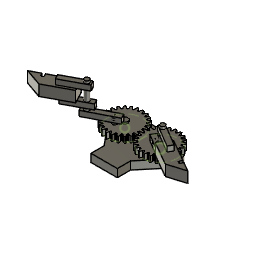
Manus Claw v1 (Autodesk Fusion 360 design; units mm, degrees)
description: Spur Gear; Module: 0.550000; Num Teeth: 24; Pressure Angle: 20.000000; Backlash: 0.00 mm
description: Spur Gear; Module: 0.5500000021653543; Num Teeth: 24; Pressure Angle: 20.0; Backlash: 0.00 mm
Autodesk Fusion 360 part; units mm, degrees
(part 1 of 11)
sketch "Sketch5" plane through (0, 0, 0) normal (0, 0, 1) x (1, 0, 0)
  line L0 (0, 0) -> (10, 0)
  line L1 (10, 0) -> (10, 5)
  line L2 (10, 5) -> (0, 5)
  line L3 (0, 5) -> (0, 0)
  line L4 (0, 5) -> (0, 10)
  line L5 (0, 10) -> (-8.1241, 19.7489)
  arc A0 (-7.2201, 22.9266) -> (-8.1241, 19.7489) centre (-6.5876, 21.0293) ccw
  line L6 (10, 5) -> (10, 10)
  line L7 (-7.2201, 22.9266) -> (-1.2199, 25.4807)
  line L8 (1.3259, 26) -> (5, 26)
  line L9 (0, 10) -> (10, 10)
  arc A1 (1.3259, 26) -> (-1.2199, 25.4807) centre (1.3259, 19.5) ccw
  line L10 (10, 10) -> (18.1241, 19.7489)
  line L11 (17.2201, 22.9266) -> (11.2199, 25.4807)
  line L12 (8.6741, 26) -> (5, 26)
  arc A2 (11.2199, 25.4807) -> (8.6741, 26) centre (8.6741, 19.5) ccw
  arc A3 (18.1241, 19.7489) -> (17.2201, 22.9266) centre (16.5876, 21.0293) ccw
  line L13 (10, 10) -> (0, 10)
  dimension "d15" = 2
  dimension "d24" = 6.5
  constraint horizontal L0
  constraint vertical L1
  constraint horizontal L2
  constraint vertical L3
  constraint coincident L0.start L3.end
  constraint perpendicular L2 L4
  constraint tangent L5 A0
  constraint horizontal L8
  constraint perpendicular L6 L9
  constraint tangent L7 A1
  constraint tangent L8 A1
  measures "d15" radius of A0
  measures "d24" radius of A1
extrude "Extrude5" add sketch "Sketch5" along normal blind 3 contours L2 L4 L6 L9 L13 | L5 A0 L7 L8 L9 A1 L10 L11 L12 A2 A3 L13 makes body 1
sketch "Sketch20" plane through (0, 0, 3) normal (0, 0, 1) x (-1, 0, 0)
  line L0 (-10, -5) -> (-10, -10)
  line L1 (-10, -10) -> (-18.1241, -19.7489)
  arc A0 (-18.1241, -19.7489) -> (-17.2201, -22.9266) centre (-16.5876, -21.0293) ccw
  line L2 (-17.2201, -22.9266) -> (-11.2199, -25.4807)
  arc A1 (-11.2199, -25.4807) -> (-8.6741, -26) centre (-8.6741, -19.5) ccw
  line L3 (-8.6741, -26) -> (-1.3259, -26)
  arc A2 (-1.3259, -26) -> (1.2199, -25.4807) centre (-1.3259, -19.5) ccw
  line L4 (1.2199, -25.4807) -> (7.2201, -22.9266)
  arc A3 (7.2201, -22.9266) -> (8.1241, -19.7489) centre (6.5876, -21.0293) ccw
  line L5 (8.1241, -19.7489) -> (0, -10)
  line L6 (0, -10) -> (0, -5)
  line L7 (0, -5) -> (-10, -5)
  line L8 (-5, -26) -> (-5, -5) construction
  circle A4 centre (1.6741, -19.5) radius 1.225
  circle A5 centre (-11.6741, -19.5) radius 1.225
  point P0 (-11.6741, -19.5)
  dimension "d136" = 2.45
  dimension "d137" = 2.45
  constraint midpoint L3 L8.start
  constraint midpoint L7 L8.end
  constraint symmetric L8 A4.centre P0
  constraint coincident P0 A5.centre
  measures "d136" diameter of A4
  measures "d137" diameter of A5
sketch "Sketch1" plane through (0, 0, 0) normal (0, 0, 1) x (1, 0, 0) in component "Spur Gear (24 teeth)"
  circle A0 centre (0, 0) radius 5.8892
  circle A1 centre (0, 0) radius 1.25
extrude "Extrude1" add sketch "Sketch1" along normal blind 2.2 separate body makes body 2 in component "Spur Gear (24 teeth)"
sketch "Sketch2" plane through (0, 0, 0) normal (0, 0, 1) x (1, 0, 0) in component "Spur Gear (24 teeth)"
  spline S0 degree 5 poles (6.182, -0.4978) (6.1847, -0.498) (6.1902, -0.4984) (6.1984, -0.4987) (6.2094, -0.4988) (6.2232, -0.4984) (6.2369, -0.4976) (6.2507, -0.4965) (6.2645, -0.4954) (6.2783, -0.4941) (6.2921, -0.4927) (6.306, -0.4912) (6.3198, -0.4895) (6.3336, -0.4877) (6.3475, -0.4857) (6.3613, -0.4835) (6.3752, -0.4811) (6.389, -0.4786) (6.4029, -0.476) (6.4168, -0.4733) (6.4306, -0.4705) (6.4445, -0.4676) (6.4583, -0.4646) (6.4722, -0.4615) (6.4861, -0.4582) (6.4999, -0.4548) (6.5138, -0.4514) (6.5277, -0.4478) (6.5415, -0.4441) (6.5554, -0.4403) (6.5693, -0.4364) (6.5831, -0.4325) (6.597, -0.4284) (6.6109, -0.4242) (6.6247, -0.42) (6.6386, -0.4156) (6.6524, -0.4112) (6.6663, -0.4067) (6.6801, -0.402) (6.694, -0.3973) (6.7078, -0.3925) (6.7216, -0.3877) (6.7355, -0.3827) (6.7493, -0.3776) (6.7631, -0.3725) (6.7769, -0.3673) (6.7907, -0.362) (6.8045, -0.3566) (6.8183, -0.3511) (6.8321, -0.3456) (6.8459, -0.3399) (6.8597, -0.3342) (6.8735, -0.3284) (6.8872, -0.3226) (6.901, -0.3166) (6.9147, -0.3106) (6.9285, -0.3045) (6.9422, -0.2983) (6.956, -0.2921) (6.9697, -0.2857) (6.9834, -0.2793) (6.9971, -0.2729) (7.0108, -0.2663) (7.0245, -0.2597) (7.0382, -0.253) (7.0519, -0.2462) (7.0655, -0.2394) (7.0792, -0.2324) (7.0928, -0.2254) (7.1064, -0.2184) (7.1201, -0.2113) (7.131, -0.2055) (7.1391, -0.2011) (7.1446, -0.1982) (7.1473, -0.1968) knots 0 0 0 0 0 0 0.01428571 0.02857143 0.04285714 0.05714286 0.07142857 0.08571429 0.1 0.11428571 0.12857143 0.14285714 0.15714286 0.17142857 0.18571429 0.2 0.21428571 0.22857143 0.24285714 0.25714286 0.27142857 0.28571429 0.3 0.31428571 0.32857143 0.34285714 0.35714286 0.37142857 0.38571429 0.4 0.41428571 0.42857143 0.44285714 0.45714286 0.47142857 0.48571429 0.5 0.51428571 0.52857143 0.54285714 0.55714286 0.57142857 0.58571429 0.6 0.61428571 0.62857143 0.64285714 0.65714286 0.67142857 0.68571429 0.7 0.71428571 0.72857143 0.74285714 0.75714286 0.77142857 0.78571429 0.8 0.81428571 0.82857143 0.84285714 0.85714286 0.87142857 0.88571429 0.9 0.91428571 0.92857143 0.94285714 0.95714286 0.97142857 0.98571429 1 1 1 1 1 1
  spline S1 degree 5 poles (6.182, 0.4978) (6.1847, 0.498) (6.1902, 0.4984) (6.1984, 0.4987) (6.2094, 0.4988) (6.2232, 0.4984) (6.2369, 0.4976) (6.2507, 0.4965) (6.2645, 0.4954) (6.2783, 0.4941) (6.2921, 0.4927) (6.306, 0.4912) (6.3198, 0.4895) (6.3336, 0.4877) (6.3475, 0.4857) (6.3613, 0.4835) (6.3752, 0.4811) (6.389, 0.4786) (6.4029, 0.476) (6.4168, 0.4733) (6.4306, 0.4705) (6.4445, 0.4676) (6.4583, 0.4646) (6.4722, 0.4615) (6.4861, 0.4582) (6.4999, 0.4548) (6.5138, 0.4514) (6.5277, 0.4478) (6.5415, 0.4441) (6.5554, 0.4403) (6.5693, 0.4364) (6.5831, 0.4325) (6.597, 0.4284) (6.6109, 0.4242) (6.6247, 0.42) (6.6386, 0.4156) (6.6524, 0.4112) (6.6663, 0.4067) (6.6801, 0.402) (6.694, 0.3973) (6.7078, 0.3925) (6.7216, 0.3877) (6.7355, 0.3827) (6.7493, 0.3776) (6.7631, 0.3725) (6.7769, 0.3673) (6.7907, 0.362) (6.8045, 0.3566) (6.8183, 0.3511) (6.8321, 0.3456) (6.8459, 0.3399) (6.8597, 0.3342) (6.8735, 0.3284) (6.8872, 0.3226) (6.901, 0.3166) (6.9147, 0.3106) (6.9285, 0.3045) (6.9422, 0.2983) (6.956, 0.2921) (6.9697, 0.2857) (6.9834, 0.2793) (6.9971, 0.2729) (7.0108, 0.2663) (7.0245, 0.2597) (7.0382, 0.253) (7.0519, 0.2462) (7.0655, 0.2394) (7.0792, 0.2324) (7.0928, 0.2254) (7.1064, 0.2184) (7.1201, 0.2113) (7.131, 0.2055) (7.1391, 0.2011) (7.1446, 0.1982) (7.1473, 0.1968) knots 0 0 0 0 0 0 0.01428571 0.02857143 0.04285714 0.05714286 0.07142857 0.08571429 0.1 0.11428571 0.12857143 0.14285714 0.15714286 0.17142857 0.18571429 0.2 0.21428571 0.22857143 0.24285714 0.25714286 0.27142857 0.28571429 0.3 0.31428571 0.32857143 0.34285714 0.35714286 0.37142857 0.38571429 0.4 0.41428571 0.42857143 0.44285714 0.45714286 0.47142857 0.48571429 0.5 0.51428571 0.52857143 0.54285714 0.55714286 0.57142857 0.58571429 0.6 0.61428571 0.62857143 0.64285714 0.65714286 0.67142857 0.68571429 0.7 0.71428571 0.72857143 0.74285714 0.75714286 0.77142857 0.78571429 0.8 0.81428571 0.82857143 0.84285714 0.85714286 0.87142857 0.88571429 0.9 0.91428571 0.92857143 0.94285714 0.95714286 0.97142857 0.98571429 1 1 1 1 1 1
  arc A0 (7.1473, -0.1968) -> (7.1473, 0.1968) centre (0, 0) ccw
  line L0 (5.8602, -0.4727) -> (6.182, -0.4978)
  line L1 (5.8602, 0.4727) -> (6.182, 0.4978)
  line L2 (5.8602, -0.4727) -> (5.8602, 0.4727)
  point P0 (6.25, -0.4966)
  point P1 (6.3185, -0.4897)
  point P2 (6.3872, -0.4789)
  point P3 (6.4561, -0.4651)
  point P4 (6.5252, -0.4484)
  point P5 (6.5943, -0.4292)
  point P6 (6.6635, -0.4075)
  point P7 (6.7328, -0.3836)
  point P8 (6.802, -0.3575)
  point P9 (6.8712, -0.3294)
  point P10 (6.9404, -0.2991)
  point P11 (7.0095, -0.2669)
  point P12 (7.0785, -0.2328)
  point P13 (6.25, 0.4966)
  point P14 (6.3185, 0.4897)
  point P15 (6.3872, 0.4789)
  point P16 (6.4561, 0.4651)
  point P17 (6.5252, 0.4484)
  point P18 (6.5943, 0.4292)
  point P19 (6.6635, 0.4075)
  point P20 (6.7328, 0.3836)
  point P21 (6.802, 0.3575)
  point P22 (6.8712, 0.3294)
  point P23 (6.9404, 0.2991)
  point P24 (7.0095, 0.2669)
  point P25 (7.0785, 0.2328)
extrude "Extrude2" add sketch "Sketch2" along normal blind 2.2 bodies 2 in component "Spur Gear (24 teeth)"
fillet "Fillet1" radius 0.25 2 edges at (5.8701, -0.4735, 1.1) (5.8701, 0.4735, 1.1) on bodies 2 in component "Spur Gear (24 teeth)"
pattern_circular "C-Pattern1" count 24 over 360 about axis through (0, 0, 0) along (0, 0, 1) of "Extrude2", "Fillet1" in component "Spur Gear (24 teeth)"
sketch "Sketch3" plane through (0, 0, 0) normal (0, 0, 1) x (1, 0, 0) in component "Spur Gear (24 teeth)"
  circle A0 centre (0, 0) radius 6.6 construction
extrude "Extrude16" add sketch "Sketch20" along normal blind 3 contours A4 | A5 bodies 1
sketch "Sketch1 (2)" plane through (0, 0, 0) normal (0, 0, 1) x (1, 0, 0) in component "Spur Gear (24 teeth) (1)"
  circle A0 centre (0, 0) radius 5.8892
  circle A1 centre (0, 0) radius 1.25
extrude "Extrude1'" add sketch "Sketch1 (2)" along normal blind 2.2 separate body makes body 3 in component "Spur Gear (24 teeth) (1)"
sketch "Sketch2 (2)" plane through (0, 0, 0) normal (0, 0, 1) x (1, 0, 0) in component "Spur Gear (24 teeth) (1)"
  spline S0 degree 5 poles (6.182, -0.4978) (6.1847, -0.498) (6.1902, -0.4984) (6.1984, -0.4987) (6.2094, -0.4988) (6.2232, -0.4984) (6.2369, -0.4976) (6.2507, -0.4965) (6.2645, -0.4954) (6.2783, -0.4941) (6.2921, -0.4927) (6.306, -0.4912) (6.3198, -0.4895) (6.3336, -0.4877) (6.3475, -0.4857) (6.3613, -0.4835) (6.3752, -0.4811) (6.389, -0.4786) (6.4029, -0.476) (6.4168, -0.4733) (6.4306, -0.4705) (6.4445, -0.4676) (6.4583, -0.4646) (6.4722, -0.4615) (6.4861, -0.4582) (6.4999, -0.4548) (6.5138, -0.4514) (6.5277, -0.4478) (6.5415, -0.4441) (6.5554, -0.4403) (6.5693, -0.4364) (6.5831, -0.4325) (6.597, -0.4284) (6.6109, -0.4242) (6.6247, -0.42) (6.6386, -0.4156) (6.6524, -0.4112) (6.6663, -0.4067) (6.6801, -0.402) (6.694, -0.3973) (6.7078, -0.3925) (6.7216, -0.3877) (6.7355, -0.3827) (6.7493, -0.3776) (6.7631, -0.3725) (6.7769, -0.3673) (6.7907, -0.362) (6.8045, -0.3566) (6.8183, -0.3511) (6.8321, -0.3456) (6.8459, -0.3399) (6.8597, -0.3342) (6.8735, -0.3284) (6.8872, -0.3226) (6.901, -0.3166) (6.9147, -0.3106) (6.9285, -0.3045) (6.9422, -0.2983) (6.956, -0.2921) (6.9697, -0.2857) (6.9834, -0.2793) (6.9971, -0.2729) (7.0108, -0.2663) (7.0245, -0.2597) (7.0382, -0.253) (7.0519, -0.2462) (7.0655, -0.2394) (7.0792, -0.2324) (7.0928, -0.2254) (7.1064, -0.2184) (7.1201, -0.2113) (7.131, -0.2055) (7.1391, -0.2011) (7.1446, -0.1982) (7.1473, -0.1968) knots 0 0 0 0 0 0 0.01428571 0.02857143 0.04285714 0.05714286 0.07142857 0.08571429 0.1 0.11428571 0.12857143 0.14285714 0.15714286 0.17142857 0.18571429 0.2 0.21428571 0.22857143 0.24285714 0.25714286 0.27142857 0.28571429 0.3 0.31428571 0.32857143 0.34285714 0.35714286 0.37142857 0.38571429 0.4 0.41428571 0.42857143 0.44285714 0.45714286 0.47142857 0.48571429 0.5 0.51428571 0.52857143 0.54285714 0.55714286 0.57142857 0.58571429 0.6 0.61428571 0.62857143 0.64285714 0.65714286 0.67142857 0.68571429 0.7 0.71428571 0.72857143 0.74285714 0.75714286 0.77142857 0.78571429 0.8 0.81428571 0.82857143 0.84285714 0.85714286 0.87142857 0.88571429 0.9 0.91428571 0.92857143 0.94285714 0.95714286 0.97142857 0.98571429 1 1 1 1 1 1
  spline S1 degree 5 poles (6.182, 0.4978) (6.1847, 0.498) (6.1902, 0.4984) (6.1984, 0.4987) (6.2094, 0.4988) (6.2232, 0.4984) (6.2369, 0.4976) (6.2507, 0.4965) (6.2645, 0.4954) (6.2783, 0.4941) (6.2921, 0.4927) (6.306, 0.4912) (6.3198, 0.4895) (6.3336, 0.4877) (6.3475, 0.4857) (6.3613, 0.4835) (6.3752, 0.4811) (6.389, 0.4786) (6.4029, 0.476) (6.4168, 0.4733) (6.4306, 0.4705) (6.4445, 0.4676) (6.4583, 0.4646) (6.4722, 0.4615) (6.4861, 0.4582) (6.4999, 0.4548) (6.5138, 0.4514) (6.5277, 0.4478) (6.5415, 0.4441) (6.5554, 0.4403) (6.5693, 0.4364) (6.5831, 0.4325) (6.597, 0.4284) (6.6109, 0.4242) (6.6247, 0.42) (6.6386, 0.4156) (6.6524, 0.4112) (6.6663, 0.4067) (6.6801, 0.402) (6.694, 0.3973) (6.7078, 0.3925) (6.7216, 0.3877) (6.7355, 0.3827) (6.7493, 0.3776) (6.7631, 0.3725) (6.7769, 0.3673) (6.7907, 0.362) (6.8045, 0.3566) (6.8183, 0.3511) (6.8321, 0.3456) (6.8459, 0.3399) (6.8597, 0.3342) (6.8735, 0.3284) (6.8872, 0.3226) (6.901, 0.3166) (6.9147, 0.3106) (6.9285, 0.3045) (6.9422, 0.2983) (6.956, 0.2921) (6.9697, 0.2857) (6.9834, 0.2793) (6.9971, 0.2729) (7.0108, 0.2663) (7.0245, 0.2597) (7.0382, 0.253) (7.0519, 0.2462) (7.0655, 0.2394) (7.0792, 0.2324) (7.0928, 0.2254) (7.1064, 0.2184) (7.1201, 0.2113) (7.131, 0.2055) (7.1391, 0.2011) (7.1446, 0.1982) (7.1473, 0.1968) knots 0 0 0 0 0 0 0.01428571 0.02857143 0.04285714 0.05714286 0.07142857 0.08571429 0.1 0.11428571 0.12857143 0.14285714 0.15714286 0.17142857 0.18571429 0.2 0.21428571 0.22857143 0.24285714 0.25714286 0.27142857 0.28571429 0.3 0.31428571 0.32857143 0.34285714 0.35714286 0.37142857 0.38571429 0.4 0.41428571 0.42857143 0.44285714 0.45714286 0.47142857 0.48571429 0.5 0.51428571 0.52857143 0.54285714 0.55714286 0.57142857 0.58571429 0.6 0.61428571 0.62857143 0.64285714 0.65714286 0.67142857 0.68571429 0.7 0.71428571 0.72857143 0.74285714 0.75714286 0.77142857 0.78571429 0.8 0.81428571 0.82857143 0.84285714 0.85714286 0.87142857 0.88571429 0.9 0.91428571 0.92857143 0.94285714 0.95714286 0.97142857 0.98571429 1 1 1 1 1 1
  arc A0 (7.1473, -0.1968) -> (7.1473, 0.1968) centre (0, 0) ccw
  line L0 (5.8602, -0.4727) -> (6.182, -0.4978)
  line L1 (5.8602, 0.4727) -> (6.182, 0.4978)
  line L2 (5.8602, -0.4727) -> (5.8602, 0.4727)
  point P0 (6.25, -0.4966)
  point P1 (6.3185, -0.4897)
  point P2 (6.3872, -0.4789)
  point P3 (6.4561, -0.4651)
  point P4 (6.5252, -0.4484)
  point P5 (6.5943, -0.4292)
  point P6 (6.6635, -0.4075)
  point P7 (6.7328, -0.3836)
  point P8 (6.802, -0.3575)
  point P9 (6.8712, -0.3294)
  point P10 (6.9404, -0.2991)
  point P11 (7.0095, -0.2669)
  point P12 (7.0785, -0.2328)
  point P13 (6.25, 0.4966)
  point P14 (6.3185, 0.4897)
  point P15 (6.3872, 0.4789)
  point P16 (6.4561, 0.4651)
  point P17 (6.5252, 0.4484)
  point P18 (6.5943, 0.4292)
  point P19 (6.6635, 0.4075)
  point P20 (6.7328, 0.3836)
  point P21 (6.802, 0.3575)
  point P22 (6.8712, 0.3294)
  point P23 (6.9404, 0.2991)
  point P24 (7.0095, 0.2669)
  point P25 (7.0785, 0.2328)
extrude "Extrude2'" add sketch "Sketch2 (2)" along normal blind 2.2 bodies 3 in component "Spur Gear (24 teeth) (1)"
fillet "Fillet1'" radius 0.25 2 edges at (5.8701, -0.4735, 1.1) (5.8701, 0.4735, 1.1) on bodies 3 in component "Spur Gear (24 teeth) (1)"
pattern_circular "C-Pattern1'" count 24 over 360 about axis through (0, 0, 0) along (0, 0, 1) of "Extrude2'", "Fillet1'" in component "Spur Gear (24 teeth) (1)"
sketch "Sketch3 (2)" plane through (0, 0, 0) normal (0, 0, 1) x (1, 0, 0) in component "Spur Gear (24 teeth) (1)"
  circle A0 centre (0, 0) radius 6.6 construction
sketch "Sketch21" plane through (30.0306, 32.9006, 5.45) normal (0, 0, 1) x (0.920765, -0.390118, 0)
  arc A0 (-5.983, -17.9856) -> (-6.0137, -17.8745) centre (-11.6741, -19.5) ccw
  arc A1 (-5.8527, -17.5684) -> (-6.0137, -17.8745) centre (-5.7734, -17.8055) ccw
  line L0 (-5.8527, -17.5684) -> (-5.7878, -17.5467)
  spline S0 degree 5 poles (-5.7878, -17.5467) (-5.7852, -17.5458) (-5.78, -17.544) (-5.7723, -17.5411) (-5.7621, -17.5369) (-5.7496, -17.5311) (-5.7373, -17.525) (-5.725, -17.5187) (-5.7127, -17.5122) (-5.7005, -17.5056) (-5.6883, -17.499) (-5.6762, -17.4922) (-5.6641, -17.4853) (-5.6521, -17.4782) (-5.6401, -17.4709) (-5.6282, -17.4635) (-5.6164, -17.4559) (-5.6046, -17.4482) (-5.5929, -17.4404) (-5.5812, -17.4326) (-5.5695, -17.4246) (-5.5579, -17.4165) (-5.5463, -17.4083) (-5.5347, -17.4) (-5.5232, -17.3916) (-5.5118, -17.3831) (-5.5004, -17.3744) (-5.489, -17.3657) (-5.4777, -17.3569) (-5.4664, -17.3481) (-5.4551, -17.3391) (-5.4439, -17.33) (-5.4327, -17.3209) (-5.4216, -17.3116) (-5.4105, -17.3023) (-5.3994, -17.2929) (-5.3884, -17.2834) (-5.3774, -17.2738) (-5.3665, -17.2642) (-5.3556, -17.2544) (-5.3447, -17.2446) (-5.3339, -17.2347) (-5.3231, -17.2247) (-5.3123, -17.2147) (-5.3016, -17.2046) (-5.2909, -17.1944) (-5.2803, -17.1841) (-5.2697, -17.1738) (-5.2591, -17.1633) (-5.2486, -17.1529) (-5.2381, -17.1423) (-5.2276, -17.1317) (-5.2172, -17.121) (-5.2068, -17.1102) (-5.1964, -17.0993) (-5.1861, -17.0884) (-5.1758, -17.0774) (-5.1656, -17.0664) (-5.1554, -17.0553) (-5.1452, -17.0441) (-5.1351, -17.0329) (-5.125, -17.0215) (-5.1149, -17.0102) (-5.1049, -16.9987) (-5.0949, -16.9872) (-5.085, -16.9756) (-5.0751, -16.964) (-5.0652, -16.9523) (-5.0554, -16.9406) (-5.0456, -16.9287) (-5.0358, -16.9168) (-5.028, -16.9073) (-5.0222, -16.9001) (-5.0183, -16.8953) (-5.0164, -16.8929) knots 0 0 0 0 0 0 0.01428571 0.02857143 0.04285714 0.05714286 0.07142857 0.08571429 0.1 0.11428571 0.12857143 0.14285714 0.15714286 0.17142857 0.18571429 0.2 0.21428571 0.22857143 0.24285714 0.25714286 0.27142857 0.28571429 0.3 0.31428571 0.32857143 0.34285714 0.35714286 0.37142857 0.38571429 0.4 0.41428571 0.42857143 0.44285714 0.45714286 0.47142857 0.48571429 0.5 0.51428571 0.52857143 0.54285714 0.55714286 0.57142857 0.58571429 0.6 0.61428571 0.62857143 0.64285714 0.65714286 0.67142857 0.68571429 0.7 0.71428571 0.72857143 0.74285714 0.75714286 0.77142857 0.78571429 0.8 0.81428571 0.82857143 0.84285714 0.85714286 0.87142857 0.88571429 0.9 0.91428571 0.92857143 0.94285714 0.95714286 0.97142857 0.98571429 1 1 1 1 1 1
  arc A2 (-5.0164, -16.8929) -> (-5.1699, -16.5306) centre (-11.6741, -19.5) ccw
  spline S1 degree 5 poles (-5.1699, -16.5306) (-5.173, -16.5303) (-5.1791, -16.5297) (-5.1884, -16.5289) (-5.2006, -16.5278) (-5.216, -16.5266) (-5.2313, -16.5254) (-5.2466, -16.5243) (-5.2618, -16.5232) (-5.2771, -16.5223) (-5.2923, -16.5213) (-5.3075, -16.5205) (-5.3227, -16.5198) (-5.3379, -16.5191) (-5.353, -16.5184) (-5.3682, -16.5179) (-5.3833, -16.5174) (-5.3984, -16.517) (-5.4134, -16.5167) (-5.4285, -16.5164) (-5.4435, -16.5163) (-5.4585, -16.5162) (-5.4734, -16.5161) (-5.4884, -16.5162) (-5.5033, -16.5163) (-5.5182, -16.5165) (-5.533, -16.5168) (-5.5479, -16.5171) (-5.5627, -16.5175) (-5.5775, -16.518) (-5.5922, -16.5186) (-5.607, -16.5193) (-5.6217, -16.52) (-5.6363, -16.5208) (-5.651, -16.5217) (-5.6656, -16.5227) (-5.6802, -16.5238) (-5.6947, -16.5249) (-5.7092, -16.5262) (-5.7237, -16.5275) (-5.7382, -16.5289) (-5.7526, -16.5304) (-5.767, -16.5319) (-5.7813, -16.5336) (-5.7956, -16.5353) (-5.8099, -16.5372) (-5.8242, -16.5391) (-5.8384, -16.5411) (-5.8525, -16.5432) (-5.8667, -16.5455) (-5.8807, -16.5478) (-5.8948, -16.5502) (-5.9088, -16.5527) (-5.9227, -16.5553) (-5.9366, -16.558) (-5.9505, -16.5609) (-5.9643, -16.5638) (-5.9781, -16.5668) (-5.9918, -16.5699) (-6.0055, -16.5732) (-6.0191, -16.5765) (-6.0326, -16.5801) (-6.0461, -16.5838) (-6.0594, -16.5877) (-6.0728, -16.5917) (-6.086, -16.5958) (-6.0992, -16.6) (-6.1124, -16.6043) (-6.1255, -16.6087) (-6.1385, -16.6133) (-6.1513, -16.6183) (-6.1614, -16.6227) (-6.1689, -16.6262) (-6.1738, -16.6287) (-6.1762, -16.6299) knots -1 -1 -1 -1 -1 -1 -0.98571429 -0.97142857 -0.95714286 -0.94285714 -0.92857143 -0.91428571 -0.9 -0.88571429 -0.87142857 -0.85714286 -0.84285714 -0.82857143 -0.81428571 -0.8 -0.78571429 -0.77142857 -0.75714286 -0.74285714 -0.72857143 -0.71428571 -0.7 -0.68571429 -0.67142857 -0.65714286 -0.64285714 -0.62857143 -0.61428571 -0.6 -0.58571429 -0.57142857 -0.55714286 -0.54285714 -0.52857143 -0.51428571 -0.5 -0.48571429 -0.47142857 -0.45714286 -0.44285714 -0.42857143 -0.41428571 -0.4 -0.38571429 -0.37142857 -0.35714286 -0.34285714 -0.32857143 -0.31428571 -0.3 -0.28571429 -0.27142857 -0.25714286 -0.24285714 -0.22857143 -0.21428571 -0.2 -0.18571429 -0.17142857 -0.15714286 -0.14285714 -0.12857143 -0.11428571 -0.1 -0.08571429 -0.07142857 -0.05714286 -0.04285714 -0.02857143 -0.01428571 0 0 0 0 0 0
  line L1 (-6.1762, -16.6299) -> (-6.237, -16.6615)
  arc A3 (-6.5689, -16.5642) -> (-6.237, -16.6615) centre (-6.3521, -16.4396) ccw
  arc A4 (-6.5689, -16.5642) -> (-6.6273, -16.4649) centre (-11.6741, -19.5) ccw
  arc A5 (-6.551, -16.1275) -> (-6.6273, -16.4649) centre (-6.4131, -16.336) ccw
  line L2 (-6.551, -16.1275) -> (-6.4939, -16.0897)
  spline S2 degree 5 poles (-6.4939, -16.0897) (-6.4916, -16.0882) (-6.4871, -16.0851) (-6.4804, -16.0803) (-6.4717, -16.0737) (-6.4611, -16.0649) (-6.4507, -16.0558) (-6.4405, -16.0464) (-6.4304, -16.037) (-6.4203, -16.0275) (-6.4102, -16.0179) (-6.4002, -16.0082) (-6.3903, -15.9984) (-6.3806, -15.9885) (-6.3709, -15.9783) (-6.3613, -15.9681) (-6.3519, -15.9577) (-6.3425, -15.9472) (-6.3331, -15.9367) (-6.3239, -15.926) (-6.3147, -15.9153) (-6.3055, -15.9045) (-6.2964, -15.8936) (-6.2874, -15.8825) (-6.2785, -15.8714) (-6.2697, -15.8603) (-6.2609, -15.849) (-6.2521, -15.8376) (-6.2435, -15.8262) (-6.2349, -15.8147) (-6.2263, -15.8031) (-6.2178, -15.7914) (-6.2094, -15.7797) (-6.201, -15.7679) (-6.1927, -15.756) (-6.1845, -15.7441) (-6.1763, -15.7321) (-6.1682, -15.72) (-6.1601, -15.7078) (-6.1521, -15.6956) (-6.1441, -15.6833) (-6.1362, -15.6709) (-6.1284, -15.6585) (-6.1206, -15.646) (-6.1128, -15.6335) (-6.1052, -15.6208) (-6.0975, -15.6082) (-6.09, -15.5954) (-6.0824, -15.5826) (-6.075, -15.5698) (-6.0676, -15.5568) (-6.0602, -15.5439) (-6.0529, -15.5308) (-6.0457, -15.5177) (-6.0385, -15.5046) (-6.0313, -15.4914) (-6.0243, -15.4781) (-6.0172, -15.4648) (-6.0103, -15.4514) (-6.0033, -15.438) (-5.9964, -15.4245) (-5.9896, -15.411) (-5.9829, -15.3974) (-5.9761, -15.3837) (-5.9695, -15.37) (-5.9629, -15.3563) (-5.9563, -15.3425) (-5.9498, -15.3286) (-5.9433, -15.3147) (-5.9369, -15.3007) (-5.9306, -15.2867) (-5.9255, -15.2755) (-5.9218, -15.267) (-5.9193, -15.2614) (-5.918, -15.2586) knots 0 0 0 0 0 0 0.01428571 0.02857143 0.04285714 0.05714286 0.07142857 0.08571429 0.1 0.11428571 0.12857143 0.14285714 0.15714286 0.17142857 0.18571429 0.2 0.21428571 0.22857143 0.24285714 0.25714286 0.27142857 0.28571429 0.3 0.31428571 0.32857143 0.34285714 0.35714286 0.37142857 0.38571429 0.4 0.41428571 0.42857143 0.44285714 0.45714286 0.47142857 0.48571429 0.5 0.51428571 0.52857143 0.54285714 0.55714286 0.57142857 0.58571429 0.6 0.61428571 0.62857143 0.64285714 0.65714286 0.67142857 0.68571429 0.7 0.71428571 0.72857143 0.74285714 0.75714286 0.77142857 0.78571429 0.8 0.81428571 0.82857143 0.84285714 0.85714286 0.87142857 0.88571429 0.9 0.91428571 0.92857143 0.94285714 0.95714286 0.97142857 0.98571429 1 1 1 1 1 1
  arc A6 (-5.918, -15.2586) -> (-6.1601, -14.9483) centre (-11.6741, -19.5) ccw
  spline S3 degree 5 poles (-6.1601, -14.9483) (-6.1631, -14.9488) (-6.1692, -14.9499) (-6.1783, -14.9515) (-6.1905, -14.9536) (-6.2056, -14.9564) (-6.2207, -14.9592) (-6.2358, -14.9621) (-6.2508, -14.965) (-6.2658, -14.968) (-6.2807, -14.9711) (-6.2956, -14.9742) (-6.3105, -14.9774) (-6.3253, -14.9807) (-6.3401, -14.984) (-6.3549, -14.9874) (-6.3696, -14.9909) (-6.3843, -14.9944) (-6.3989, -14.998) (-6.4135, -15.0016) (-6.428, -15.0053) (-6.4425, -15.0091) (-6.457, -15.0129) (-6.4714, -15.0168) (-6.4858, -15.0208) (-6.5001, -15.0249) (-6.5144, -15.029) (-6.5287, -15.0332) (-6.5429, -15.0374) (-6.557, -15.0417) (-6.5711, -15.0461) (-6.5852, -15.0505) (-6.5992, -15.0551) (-6.6131, -15.0597) (-6.627, -15.0643) (-6.6409, -15.069) (-6.6547, -15.0738) (-6.6685, -15.0787) (-6.6822, -15.0837) (-6.6958, -15.0887) (-6.7094, -15.0938) (-6.723, -15.0989) (-6.7365, -15.1042) (-6.7499, -15.1095) (-6.7633, -15.1149) (-6.7766, -15.1204) (-6.7898, -15.1259) (-6.803, -15.1315) (-6.8162, -15.1373) (-6.8292, -15.143) (-6.8422, -15.1489) (-6.8552, -15.1549) (-6.868, -15.1609) (-6.8808, -15.1671) (-6.8936, -15.1733) (-6.9062, -15.1796) (-6.9188, -15.186) (-6.9313, -15.1925) (-6.9438, -15.1991) (-6.9561, -15.2057) (-6.9684, -15.2125) (-6.9806, -15.2194) (-6.9926, -15.2265) (-7.0045, -15.2337) (-7.0164, -15.241) (-7.0281, -15.2484) (-7.0398, -15.2559) (-7.0514, -15.2635) (-7.0629, -15.2711) (-7.0743, -15.279) (-7.0854, -15.2871) (-7.094, -15.2939) (-7.1002, -15.2993) (-7.1043, -15.3029) (-7.1064, -15.3048) knots -1 -1 -1 -1 -1 -1 -0.98571429 -0.97142857 -0.95714286 -0.94285714 -0.92857143 -0.91428571 -0.9 -0.88571429 -0.87142857 -0.85714286 -0.84285714 -0.82857143 -0.81428571 -0.8 -0.78571429 -0.77142857 -0.75714286 -0.74285714 -0.72857143 -0.71428571 -0.7 -0.68571429 -0.67142857 -0.65714286 -0.64285714 -0.62857143 -0.61428571 -0.6 -0.58571429 -0.57142857 -0.55714286 -0.54285714 -0.52857143 -0.51428571 -0.5 -0.48571429 -0.47142857 -0.45714286 -0.44285714 -0.42857143 -0.41428571 -0.4 -0.38571429 -0.37142857 -0.35714286 -0.34285714 -0.32857143 -0.31428571 -0.3 -0.28571429 -0.27142857 -0.25714286 -0.24285714 -0.22857143 -0.21428571 -0.2 -0.18571429 -0.17142857 -0.15714286 -0.14285714 -0.12857143 -0.11428571 -0.1 -0.08571429 -0.07142857 -0.05714286 -0.04285714 -0.02857143 -0.01428571 0 0 0 0 0 0
  line L3 (-7.1064, -15.3048) -> (-7.1569, -15.351)
  arc A7 (-7.5027, -15.3429) -> (-7.1569, -15.351) centre (-7.3256, -15.1664) ccw
  arc A8 (-7.5027, -15.3429) -> (-7.5848, -15.2621) centre (-11.6741, -19.5) ccw
  arc A9 (-7.5985, -14.9165) -> (-7.5848, -15.2621) centre (-7.4112, -15.0822) ccw
  line L4 (-7.5985, -14.9165) -> (-7.5531, -14.8652)
  spline S4 degree 5 poles (-7.5531, -14.8652) (-7.5513, -14.8631) (-7.5477, -14.859) (-7.5424, -14.8526) (-7.5357, -14.8439) (-7.5278, -14.8327) (-7.5201, -14.8212) (-7.5127, -14.8096) (-7.5053, -14.7978) (-7.498, -14.786) (-7.4908, -14.7742) (-7.4837, -14.7622) (-7.4767, -14.7502) (-7.4698, -14.738) (-7.4631, -14.7258) (-7.4565, -14.7134) (-7.45, -14.7009) (-7.4437, -14.6884) (-7.4374, -14.6757) (-7.4312, -14.663) (-7.4251, -14.6503) (-7.419, -14.6375) (-7.4131, -14.6246) (-7.4073, -14.6116) (-7.4015, -14.5986) (-7.3958, -14.5855) (-7.3903, -14.5723) (-7.3848, -14.5591) (-7.3794, -14.5458) (-7.374, -14.5325) (-7.3688, -14.5191) (-7.3636, -14.5056) (-7.3585, -14.4921) (-7.3535, -14.4785) (-7.3485, -14.4649) (-7.3436, -14.4512) (-7.3388, -14.4375) (-7.3341, -14.4237) (-7.3295, -14.4099) (-7.3249, -14.396) (-7.3204, -14.3821) (-7.3159, -14.3681) (-7.3116, -14.354) (-7.3073, -14.34) (-7.3031, -14.3258) (-7.2989, -14.3117) (-7.2948, -14.2974) (-7.2908, -14.2832) (-7.2869, -14.2689) (-7.283, -14.2545) (-7.2792, -14.2401) (-7.2754, -14.2257) (-7.2718, -14.2112) (-7.2682, -14.1967) (-7.2646, -14.1821) (-7.2611, -14.1675) (-7.2577, -14.1529) (-7.2544, -14.1382) (-7.2511, -14.1234) (-7.2479, -14.1087) (-7.2447, -14.0939) (-7.2416, -14.079) (-7.2386, -14.0641) (-7.2357, -14.0492) (-7.2328, -14.0343) (-7.2299, -14.0193) (-7.2272, -14.0042) (-7.2245, -13.9892) (-7.2218, -13.9741) (-7.2193, -13.9589) (-7.2168, -13.9438) (-7.2148, -13.9316) (-7.2134, -13.9225) (-7.2124, -13.9164) (-7.2119, -13.9133) knots 0 0 0 0 0 0 0.01428571 0.02857143 0.04285714 0.05714286 0.07142857 0.08571429 0.1 0.11428571 0.12857143 0.14285714 0.15714286 0.17142857 0.18571429 0.2 0.21428571 0.22857143 0.24285714 0.25714286 0.27142857 0.28571429 0.3 0.31428571 0.32857143 0.34285714 0.35714286 0.37142857 0.38571429 0.4 0.41428571 0.42857143 0.44285714 0.45714286 0.47142857 0.48571429 0.5 0.51428571 0.52857143 0.54285714 0.55714286 0.57142857 0.58571429 0.6 0.61428571 0.62857143 0.64285714 0.65714286 0.67142857 0.68571429 0.7 0.71428571 0.72857143 0.74285714 0.75714286 0.77142857 0.78571429 0.8 0.81428571 0.82857143 0.84285714 0.85714286 0.87142857 0.88571429 0.9 0.91428571 0.92857143 0.94285714 0.95714286 0.97142857 0.98571429 1 1 1 1 1 1
  arc A10 (-7.2119, -13.9133) -> (-7.526, -13.6763) centre (-11.6741, -19.5) ccw
  spline S5 degree 5 poles (-7.526, -13.6763) (-7.5288, -13.6776) (-7.5345, -13.6802) (-7.5428, -13.684) (-7.554, -13.6893) (-7.5679, -13.6958) (-7.5818, -13.7025) (-7.5956, -13.7092) (-7.6093, -13.7159) (-7.623, -13.7227) (-7.6366, -13.7295) (-7.6502, -13.7364) (-7.6638, -13.7433) (-7.6773, -13.7503) (-7.6907, -13.7574) (-7.7041, -13.7644) (-7.7174, -13.7716) (-7.7306, -13.7788) (-7.7438, -13.786) (-7.757, -13.7933) (-7.7701, -13.8007) (-7.7831, -13.8081) (-7.7961, -13.8155) (-7.809, -13.823) (-7.8219, -13.8306) (-7.8347, -13.8382) (-7.8474, -13.8459) (-7.8601, -13.8536) (-7.8727, -13.8614) (-7.8853, -13.8692) (-7.8977, -13.8771) (-7.9102, -13.885) (-7.9225, -13.893) (-7.9348, -13.9011) (-7.9471, -13.9092) (-7.9592, -13.9173) (-7.9713, -13.9255) (-7.9833, -13.9338) (-7.9953, -13.9421) (-8.0072, -13.9505) (-8.019, -13.9589) (-8.0308, -13.9674) (-8.0424, -13.976) (-8.054, -13.9846) (-8.0655, -13.9933) (-8.077, -14.002) (-8.0884, -14.0108) (-8.0996, -14.0197) (-8.1109, -14.0286) (-8.122, -14.0375) (-8.133, -14.0466) (-8.144, -14.0557) (-8.1548, -14.0649) (-8.1656, -14.0741) (-8.1763, -14.0834) (-8.1869, -14.0928) (-8.1974, -14.1022) (-8.2078, -14.1117) (-8.2181, -14.1213) (-8.2283, -14.131) (-8.2384, -14.1407) (-8.2484, -14.1505) (-8.2582, -14.1605) (-8.2678, -14.1705) (-8.2774, -14.1806) (-8.2868, -14.1908) (-8.2961, -14.2011) (-8.3054, -14.2114) (-8.3145, -14.2217) (-8.3235, -14.2323) (-8.3321, -14.243) (-8.3387, -14.2518) (-8.3433, -14.2586) (-8.3463, -14.2632) (-8.3478, -14.2655) knots -1 -1 -1 -1 -1 -1 -0.98571429 -0.97142857 -0.95714286 -0.94285714 -0.92857143 -0.91428571 -0.9 -0.88571429 -0.87142857 -0.85714286 -0.84285714 -0.82857143 -0.81428571 -0.8 -0.78571429 -0.77142857 -0.75714286 -0.74285714 -0.72857143 -0.71428571 -0.7 -0.68571429 -0.67142857 -0.65714286 -0.64285714 -0.62857143 -0.61428571 -0.6 -0.58571429 -0.57142857 -0.55714286 -0.54285714 -0.52857143 -0.51428571 -0.5 -0.48571429 -0.47142857 -0.45714286 -0.44285714 -0.42857143 -0.41428571 -0.4 -0.38571429 -0.37142857 -0.35714286 -0.34285714 -0.32857143 -0.31428571 -0.3 -0.28571429 -0.27142857 -0.25714286 -0.24285714 -0.22857143 -0.21428571 -0.2 -0.18571429 -0.17142857 -0.15714286 -0.14285714 -0.12857143 -0.11428571 -0.1 -0.08571429 -0.07142857 -0.05714286 -0.04285714 -0.02857143 -0.01428571 0 0 0 0 0 0
  line L5 (-8.3478, -14.2655) -> (-8.3847, -14.3232)
  arc A11 (-8.7207, -14.4049) -> (-8.3847, -14.3232) centre (-8.5954, -14.1886) ccw
  arc A12 (-8.7207, -14.4049) -> (-8.821, -14.3481) centre (-11.6741, -19.5) ccw
  arc A13 (-8.9236, -14.0178) -> (-8.821, -14.3481) centre (-8.6999, -14.1294) ccw
  line L6 (-8.9236, -14.0178) -> (-8.8931, -13.9565)
  spline S6 degree 5 poles (-8.8931, -13.9565) (-8.8918, -13.9541) (-8.8895, -13.9491) (-8.886, -13.9416) (-8.8818, -13.9315) (-8.8771, -13.9186) (-8.8727, -13.9055) (-8.8685, -13.8923) (-8.8644, -13.8791) (-8.8604, -13.8658) (-8.8565, -13.8525) (-8.8527, -13.8391) (-8.849, -13.8256) (-8.8455, -13.8121) (-8.8422, -13.7985) (-8.8391, -13.7849) (-8.836, -13.7712) (-8.8332, -13.7574) (-8.8304, -13.7436) (-8.8277, -13.7297) (-8.825, -13.7158) (-8.8225, -13.7019) (-8.8201, -13.6879) (-8.8179, -13.6738) (-8.8157, -13.6598) (-8.8136, -13.6456) (-8.8116, -13.6315) (-8.8097, -13.6173) (-8.8079, -13.6031) (-8.8062, -13.5888) (-8.8046, -13.5745) (-8.8031, -13.5601) (-8.8017, -13.5458) (-8.8003, -13.5314) (-8.7991, -13.5169) (-8.7979, -13.5024) (-8.7968, -13.4879) (-8.7958, -13.4734) (-8.7949, -13.4588) (-8.7941, -13.4442) (-8.7934, -13.4296) (-8.7927, -13.415) (-8.7921, -13.4003) (-8.7916, -13.3856) (-8.7912, -13.3708) (-8.7908, -13.3561) (-8.7906, -13.3413) (-8.7904, -13.3265) (-8.7903, -13.3116) (-8.7902, -13.2967) (-8.7903, -13.2819) (-8.7904, -13.2669) (-8.7906, -13.252) (-8.7909, -13.237) (-8.7912, -13.222) (-8.7917, -13.207) (-8.7921, -13.192) (-8.7927, -13.177) (-8.7934, -13.1619) (-8.7941, -13.1468) (-8.7949, -13.1317) (-8.7957, -13.1165) (-8.7967, -13.1014) (-8.7977, -13.0862) (-8.7987, -13.071) (-8.7999, -13.0558) (-8.8011, -13.0405) (-8.8024, -13.0253) (-8.8038, -13.01) (-8.8052, -12.9947) (-8.8067, -12.9794) (-8.808, -12.9672) (-8.8089, -12.958) (-8.8096, -12.9518) (-8.8099, -12.9488) knots 0 0 0 0 0 0 0.01428571 0.02857143 0.04285714 0.05714286 0.07142857 0.08571429 0.1 0.11428571 0.12857143 0.14285714 0.15714286 0.17142857 0.18571429 0.2 0.21428571 0.22857143 0.24285714 0.25714286 0.27142857 0.28571429 0.3 0.31428571 0.32857143 0.34285714 0.35714286 0.37142857 0.38571429 0.4 0.41428571 0.42857143 0.44285714 0.45714286 0.47142857 0.48571429 0.5 0.51428571 0.52857143 0.54285714 0.55714286 0.57142857 0.58571429 0.6 0.61428571 0.62857143 0.64285714 0.65714286 0.67142857 0.68571429 0.7 0.71428571 0.72857143 0.74285714 0.75714286 0.77142857 0.78571429 0.8 0.81428571 0.82857143 0.84285714 0.85714286 0.87142857 0.88571429 0.9 0.91428571 0.92857143 0.94285714 0.95714286 0.97142857 0.98571429 1 1 1 1 1 1
  arc A14 (-8.8099, -12.9488) -> (-9.1747, -12.8011) centre (-11.6741, -19.5) ccw
  spline S7 degree 5 poles (-9.1747, -12.8011) (-9.1771, -12.8031) (-9.1818, -12.807) (-9.1889, -12.813) (-9.1983, -12.8209) (-9.2101, -12.8308) (-9.2217, -12.8408) (-9.2333, -12.8509) (-9.2449, -12.8609) (-9.2563, -12.871) (-9.2677, -12.8811) (-9.2791, -12.8913) (-9.2904, -12.9015) (-9.3016, -12.9118) (-9.3127, -12.922) (-9.3238, -12.9323) (-9.3348, -12.9427) (-9.3458, -12.9531) (-9.3567, -12.9635) (-9.3675, -12.9739) (-9.3782, -12.9844) (-9.3889, -12.995) (-9.3995, -13.0055) (-9.41, -13.0161) (-9.4205, -13.0267) (-9.4309, -13.0374) (-9.4412, -13.0481) (-9.4514, -13.0589) (-9.4616, -13.0696) (-9.4717, -13.0804) (-9.4817, -13.0913) (-9.4917, -13.1022) (-9.5016, -13.1131) (-9.5114, -13.124) (-9.5211, -13.135) (-9.5307, -13.1461) (-9.5403, -13.1571) (-9.5497, -13.1682) (-9.5591, -13.1794) (-9.5685, -13.1905) (-9.5777, -13.2017) (-9.5868, -13.213) (-9.5959, -13.2243) (-9.6049, -13.2356) (-9.6137, -13.247) (-9.6225, -13.2583) (-9.6312, -13.2698) (-9.6399, -13.2813) (-9.6484, -13.2928) (-9.6568, -13.3043) (-9.6651, -13.3159) (-9.6734, -13.3275) (-9.6815, -13.3392) (-9.6895, -13.3509) (-9.6974, -13.3627) (-9.7052, -13.3745) (-9.7129, -13.3863) (-9.7205, -13.3982) (-9.728, -13.4101) (-9.7354, -13.4221) (-9.7426, -13.4341) (-9.7497, -13.4461) (-9.7566, -13.4583) (-9.7633, -13.4705) (-9.7699, -13.4827) (-9.7763, -13.495) (-9.7827, -13.5073) (-9.789, -13.5197) (-9.7951, -13.5321) (-9.801, -13.5445) (-9.8066, -13.5571) (-9.8106, -13.5673) (-9.8134, -13.5751) (-9.8151, -13.5803) (-9.816, -13.5829) knots -1 -1 -1 -1 -1 -1 -0.98571429 -0.97142857 -0.95714286 -0.94285714 -0.92857143 -0.91428571 -0.9 -0.88571429 -0.87142857 -0.85714286 -0.84285714 -0.82857143 -0.81428571 -0.8 -0.78571429 -0.77142857 -0.75714286 -0.74285714 -0.72857143 -0.71428571 -0.7 -0.68571429 -0.67142857 -0.65714286 -0.64285714 -0.62857143 -0.61428571 -0.6 -0.58571429 -0.57142857 -0.55714286 -0.54285714 -0.52857143 -0.51428571 -0.5 -0.48571429 -0.47142857 -0.45714286 -0.44285714 -0.42857143 -0.41428571 -0.4 -0.38571429 -0.37142857 -0.35714286 -0.34285714 -0.32857143 -0.31428571 -0.3 -0.28571429 -0.27142857 -0.25714286 -0.24285714 -0.22857143 -0.21428571 -0.2 -0.18571429 -0.17142857 -0.15714286 -0.14285714 -0.12857143 -0.11428571 -0.1 -0.08571429 -0.07142857 -0.05714286 -0.04285714 -0.02857143 -0.01428571 0 0 0 0 0 0
  line L7 (-9.816, -13.5829) -> (-9.8366, -13.6482)
  arc A15 (-10.1401, -13.8141) -> (-9.8366, -13.6482) centre (-10.075, -13.5727) ccw
  arc A16 (-10.1401, -13.8141) -> (-10.2517, -13.7852) centre (-11.6741, -19.5) ccw
  arc A17 (-10.4362, -13.4927) -> (-10.2517, -13.7852) centre (-10.1913, -13.5426) ccw
  line L8 (-10.4362, -13.4927) -> (-10.4226, -13.4256)
  spline S8 degree 5 poles (-10.4226, -13.4256) (-10.422, -13.4229) (-10.421, -13.4175) (-10.4197, -13.4094) (-10.4182, -13.3985) (-10.417, -13.3848) (-10.4161, -13.371) (-10.4154, -13.3572) (-10.4149, -13.3434) (-10.4145, -13.3295) (-10.4142, -13.3156) (-10.414, -13.3017) (-10.4139, -13.2878) (-10.4141, -13.2738) (-10.4144, -13.2599) (-10.4149, -13.2458) (-10.4155, -13.2318) (-10.4163, -13.2178) (-10.4171, -13.2037) (-10.4181, -13.1896) (-10.4192, -13.1755) (-10.4204, -13.1614) (-10.4217, -13.1473) (-10.4231, -13.1331) (-10.4246, -13.1189) (-10.4263, -13.1048) (-10.428, -13.0906) (-10.4299, -13.0764) (-10.4318, -13.0622) (-10.4339, -13.0479) (-10.436, -13.0337) (-10.4383, -13.0195) (-10.4406, -13.0052) (-10.4431, -12.9909) (-10.4456, -12.9767) (-10.4482, -12.9624) (-10.4509, -12.9481) (-10.4537, -12.9338) (-10.4566, -12.9195) (-10.4596, -12.9052) (-10.4626, -12.8909) (-10.4658, -12.8765) (-10.469, -12.8622) (-10.4724, -12.8479) (-10.4758, -12.8335) (-10.4793, -12.8192) (-10.4828, -12.8048) (-10.4865, -12.7904) (-10.4902, -12.7761) (-10.494, -12.7617) (-10.4979, -12.7473) (-10.5019, -12.733) (-10.506, -12.7186) (-10.5101, -12.7042) (-10.5143, -12.6898) (-10.5186, -12.6754) (-10.523, -12.661) (-10.5274, -12.6466) (-10.5319, -12.6322) (-10.5365, -12.6178) (-10.5412, -12.6034) (-10.546, -12.5891) (-10.5508, -12.5747) (-10.5557, -12.5603) (-10.5607, -12.5459) (-10.5657, -12.5315) (-10.5708, -12.5171) (-10.576, -12.5027) (-10.5813, -12.4883) (-10.5866, -12.4739) (-10.5921, -12.4595) (-10.5964, -12.4479) (-10.5998, -12.4393) (-10.602, -12.4336) (-10.6031, -12.4307) knots 0 0 0 0 0 0 0.01428571 0.02857143 0.04285714 0.05714286 0.07142857 0.08571429 0.1 0.11428571 0.12857143 0.14285714 0.15714286 0.17142857 0.18571429 0.2 0.21428571 0.22857143 0.24285714 0.25714286 0.27142857 0.28571429 0.3 0.31428571 0.32857143 0.34285714 0.35714286 0.37142857 0.38571429 0.4 0.41428571 0.42857143 0.44285714 0.45714286 0.47142857 0.48571429 0.5 0.51428571 0.52857143 0.54285714 0.55714286 0.57142857 0.58571429 0.6 0.61428571 0.62857143 0.64285714 0.65714286 0.67142857 0.68571429 0.7 0.71428571 0.72857143 0.74285714 0.75714286 0.77142857 0.78571429 0.8 0.81428571 0.82857143 0.84285714 0.85714286 0.87142857 0.88571429 0.9 0.91428571 0.92857143 0.94285714 0.95714286 0.97142857 0.98571429 1 1 1 1 1 1
  arc A18 (-10.6031, -12.4307) -> (-10.9936, -12.3825) centre (-11.6741, -19.5) ccw
  spline S9 degree 5 poles (-10.9936, -12.3825) (-10.9954, -12.385) (-10.999, -12.39) (-11.0043, -12.3976) (-11.0114, -12.4077) (-11.0201, -12.4203) (-11.0288, -12.433) (-11.0374, -12.4457) (-11.046, -12.4584) (-11.0544, -12.4711) (-11.0628, -12.4839) (-11.0711, -12.4966) (-11.0794, -12.5094) (-11.0876, -12.5222) (-11.0957, -12.535) (-11.1037, -12.5478) (-11.1117, -12.5607) (-11.1196, -12.5735) (-11.1274, -12.5864) (-11.1351, -12.5993) (-11.1428, -12.6122) (-11.1504, -12.6251) (-11.1579, -12.6381) (-11.1653, -12.6511) (-11.1727, -12.664) (-11.18, -12.677) (-11.1872, -12.69) (-11.1943, -12.7031) (-11.2013, -12.7161) (-11.2083, -12.7292) (-11.2151, -12.7422) (-11.2219, -12.7553) (-11.2286, -12.7684) (-11.2353, -12.7815) (-11.2418, -12.7947) (-11.2483, -12.8078) (-11.2546, -12.821) (-11.2609, -12.8341) (-11.2671, -12.8473) (-11.2732, -12.8605) (-11.2792, -12.8737) (-11.2852, -12.887) (-11.291, -12.9002) (-11.2967, -12.9135) (-11.3024, -12.9267) (-11.3079, -12.94) (-11.3134, -12.9533) (-11.3187, -12.9666) (-11.324, -12.98) (-11.3291, -12.9933) (-11.3342, -13.0067) (-11.3391, -13.02) (-11.3439, -13.0334) (-11.3486, -13.0468) (-11.3532, -13.0602) (-11.3577, -13.0736) (-11.362, -13.087) (-11.3663, -13.1005) (-11.3705, -13.1139) (-11.3745, -13.1274) (-11.3784, -13.1408) (-11.3821, -13.1543) (-11.3856, -13.1678) (-11.3889, -13.1814) (-11.3921, -13.1949) (-11.3952, -13.2084) (-11.3982, -13.222) (-11.401, -13.2355) (-11.4038, -13.2491) (-11.4063, -13.2627) (-11.4084, -13.2763) (-11.4096, -13.2872) (-11.4103, -13.2954) (-11.4106, -13.3009) (-11.4107, -13.3036) knots -1 -1 -1 -1 -1 -1 -0.98571429 -0.97142857 -0.95714286 -0.94285714 -0.92857143 -0.91428571 -0.9 -0.88571429 -0.87142857 -0.85714286 -0.84285714 -0.82857143 -0.81428571 -0.8 -0.78571429 -0.77142857 -0.75714286 -0.74285714 -0.72857143 -0.71428571 -0.7 -0.68571429 -0.67142857 -0.65714286 -0.64285714 -0.62857143 -0.61428571 -0.6 -0.58571429 -0.57142857 -0.55714286 -0.54285714 -0.52857143 -0.51428571 -0.5 -0.48571429 -0.47142857 -0.45714286 -0.44285714 -0.42857143 -0.41428571 -0.4 -0.38571429 -0.37142857 -0.35714286 -0.34285714 -0.32857143 -0.31428571 -0.3 -0.28571429 -0.27142857 -0.25714286 -0.24285714 -0.22857143 -0.21428571 -0.2 -0.18571429 -0.17142857 -0.15714286 -0.14285714 -0.12857143 -0.11428571 -0.1 -0.08571429 -0.07142857 -0.05714286 -0.04285714 -0.02857143 -0.01428571 0 0 0 0 0 0
  line L9 (-11.4107, -13.3036) -> (-11.4138, -13.372)
  arc A19 (-11.664, -13.6108) -> (-11.4138, -13.372) centre (-11.6636, -13.3608) ccw
  arc A20 (-11.664, -13.6108) -> (-11.7792, -13.6117) centre (-11.6741, -19.5) ccw
  arc A21 (-12.0332, -13.377) -> (-11.7792, -13.6117) centre (-11.7837, -13.3618) ccw
  line L10 (-12.0332, -13.377) -> (-12.0374, -13.3087)
  spline S10 degree 5 poles (-12.0374, -13.3087) (-12.0376, -13.3059) (-12.038, -13.3005) (-12.0388, -13.2923) (-12.0402, -13.2814) (-12.0425, -13.2678) (-12.0452, -13.2543) (-12.0482, -13.2408) (-12.0513, -13.2273) (-12.0545, -13.2138) (-12.0577, -13.2003) (-12.0611, -13.1868) (-12.0647, -13.1733) (-12.0684, -13.1599) (-12.0724, -13.1464) (-12.0765, -13.133) (-12.0807, -13.1196) (-12.0851, -13.1063) (-12.0896, -13.0929) (-12.0942, -13.0795) (-12.0989, -13.0662) (-12.1037, -13.0529) (-12.1086, -13.0396) (-12.1136, -13.0263) (-12.1187, -13.013) (-12.124, -12.9997) (-12.1294, -12.9865) (-12.1348, -12.9732) (-12.1404, -12.96) (-12.1461, -12.9468) (-12.1518, -12.9336) (-12.1577, -12.9204) (-12.1636, -12.9073) (-12.1697, -12.8941) (-12.1758, -12.881) (-12.182, -12.8679) (-12.1884, -12.8548) (-12.1948, -12.8417) (-12.2013, -12.8286) (-12.2078, -12.8155) (-12.2145, -12.8025) (-12.2213, -12.7895) (-12.2281, -12.7765) (-12.235, -12.7635) (-12.242, -12.7505) (-12.2491, -12.7375) (-12.2563, -12.7246) (-12.2635, -12.7117) (-12.2708, -12.6988) (-12.2782, -12.6859) (-12.2857, -12.673) (-12.2933, -12.6601) (-12.3009, -12.6473) (-12.3086, -12.6345) (-12.3164, -12.6217) (-12.3243, -12.6089) (-12.3323, -12.5961) (-12.3403, -12.5834) (-12.3484, -12.5706) (-12.3565, -12.5579) (-12.3648, -12.5452) (-12.3731, -12.5325) (-12.3815, -12.5199) (-12.3899, -12.5072) (-12.3985, -12.4946) (-12.4071, -12.482) (-12.4158, -12.4694) (-12.4245, -12.4569) (-12.4333, -12.4443) (-12.4422, -12.4318) (-12.4511, -12.4193) (-12.4584, -12.4093) (-12.4638, -12.4018) (-12.4675, -12.3968) (-12.4693, -12.3944) knots 0 0 0 0 0 0 0.01428571 0.02857143 0.04285714 0.05714286 0.07142857 0.08571429 0.1 0.11428571 0.12857143 0.14285714 0.15714286 0.17142857 0.18571429 0.2 0.21428571 0.22857143 0.24285714 0.25714286 0.27142857 0.28571429 0.3 0.31428571 0.32857143 0.34285714 0.35714286 0.37142857 0.38571429 0.4 0.41428571 0.42857143 0.44285714 0.45714286 0.47142857 0.48571429 0.5 0.51428571 0.52857143 0.54285714 0.55714286 0.57142857 0.58571429 0.6 0.61428571 0.62857143 0.64285714 0.65714286 0.67142857 0.68571429 0.7 0.71428571 0.72857143 0.74285714 0.75714286 0.77142857 0.78571429 0.8 0.81428571 0.82857143 0.84285714 0.85714286 0.87142857 0.88571429 0.9 0.91428571 0.92857143 0.94285714 0.95714286 0.97142857 0.98571429 1 1 1 1 1 1
  arc A22 (-12.4693, -12.3944) -> (-12.859, -12.4489) centre (-11.6741, -19.5) ccw
  spline S11 degree 5 poles (-12.859, -12.4489) (-12.8601, -12.4518) (-12.8622, -12.4575) (-12.8654, -12.4662) (-12.8696, -12.4778) (-12.8748, -12.4923) (-12.8799, -12.5068) (-12.8849, -12.5213) (-12.8899, -12.5357) (-12.8947, -12.5502) (-12.8996, -12.5647) (-12.9043, -12.5792) (-12.909, -12.5937) (-12.9136, -12.6081) (-12.9181, -12.6226) (-12.9225, -12.6371) (-12.9269, -12.6515) (-12.9312, -12.666) (-12.9354, -12.6805) (-12.9395, -12.6949) (-12.9436, -12.7094) (-12.9476, -12.7238) (-12.9515, -12.7383) (-12.9553, -12.7527) (-12.959, -12.7672) (-12.9627, -12.7816) (-12.9663, -12.796) (-12.9698, -12.8105) (-12.9732, -12.8249) (-12.9766, -12.8393) (-12.9798, -12.8537) (-12.983, -12.8681) (-12.9861, -12.8825) (-12.9891, -12.8969) (-12.992, -12.9112) (-12.9948, -12.9256) (-12.9976, -12.94) (-13.0002, -12.9543) (-13.0028, -12.9687) (-13.0053, -12.983) (-13.0077, -12.9973) (-13.01, -13.0116) (-13.0122, -13.0259) (-13.0143, -13.0402) (-13.0163, -13.0545) (-13.0182, -13.0688) (-13.02, -13.083) (-13.0218, -13.0973) (-13.0234, -13.1115) (-13.0249, -13.1257) (-13.0263, -13.1399) (-13.0277, -13.1541) (-13.0288, -13.1683) (-13.0299, -13.1824) (-13.0309, -13.1965) (-13.0317, -13.2107) (-13.0325, -13.2248) (-13.0331, -13.2388) (-13.0337, -13.2529) (-13.0341, -13.267) (-13.0343, -13.281) (-13.0344, -13.295) (-13.0343, -13.3089) (-13.0341, -13.3229) (-13.0336, -13.3368) (-13.0331, -13.3506) (-13.0324, -13.3645) (-13.0317, -13.3783) (-13.0308, -13.3921) (-13.0297, -13.4059) (-13.0282, -13.4195) (-13.0266, -13.4304) (-13.0251, -13.4385) (-13.024, -13.4439) (-13.0234, -13.4466) knots -1 -1 -1 -1 -1 -1 -0.98571429 -0.97142857 -0.95714286 -0.94285714 -0.92857143 -0.91428571 -0.9 -0.88571429 -0.87142857 -0.85714286 -0.84285714 -0.82857143 -0.81428571 -0.8 -0.78571429 -0.77142857 -0.75714286 -0.74285714 -0.72857143 -0.71428571 -0.7 -0.68571429 -0.67142857 -0.65714286 -0.64285714 -0.62857143 -0.61428571 -0.6 -0.58571429 -0.57142857 -0.55714286 -0.54285714 -0.52857143 -0.51428571 -0.5 -0.48571429 -0.47142857 -0.45714286 -0.44285714 -0.42857143 -0.41428571 -0.4 -0.38571429 -0.37142857 -0.35714286 -0.34285714 -0.32857143 -0.31428571 -0.3 -0.28571429 -0.27142857 -0.25714286 -0.24285714 -0.22857143 -0.21428571 -0.2 -0.18571429 -0.17142857 -0.15714286 -0.14285714 -0.12857143 -0.11428571 -0.1 -0.08571429 -0.07142857 -0.05714286 -0.04285714 -0.02857143 -0.01428571 0 0 0 0 0 0
  line L11 (-13.0234, -13.4466) -> (-13.0087, -13.5135)
  arc A23 (-13.1886, -13.8088) -> (-13.0087, -13.5135) centre (-13.2529, -13.5673) ccw
  arc A24 (-13.1886, -13.8088) -> (-13.2996, -13.8396) centre (-11.6741, -19.5) ccw
  arc A25 (-13.6057, -13.6786) -> (-13.2996, -13.8396) centre (-13.3686, -13.5993) ccw
  line L12 (-13.6057, -13.6786) -> (-13.6275, -13.6137)
  spline S12 degree 5 poles (-13.6275, -13.6137) (-13.6283, -13.6111) (-13.6301, -13.6059) (-13.633, -13.5982) (-13.6372, -13.588) (-13.643, -13.5755) (-13.6491, -13.5631) (-13.6555, -13.5508) (-13.6619, -13.5386) (-13.6685, -13.5264) (-13.6752, -13.5142) (-13.6819, -13.5021) (-13.6889, -13.49) (-13.696, -13.4779) (-13.7032, -13.466) (-13.7106, -13.4541) (-13.7182, -13.4423) (-13.7259, -13.4305) (-13.7337, -13.4187) (-13.7416, -13.407) (-13.7496, -13.3953) (-13.7577, -13.3837) (-13.7659, -13.3721) (-13.7742, -13.3606) (-13.7826, -13.3491) (-13.7911, -13.3376) (-13.7997, -13.3262) (-13.8084, -13.3149) (-13.8172, -13.3035) (-13.8261, -13.2922) (-13.8351, -13.281) (-13.8441, -13.2698) (-13.8533, -13.2586) (-13.8625, -13.2474) (-13.8718, -13.2364) (-13.8813, -13.2253) (-13.8907, -13.2143) (-13.9003, -13.2033) (-13.91, -13.1923) (-13.9197, -13.1814) (-13.9295, -13.1706) (-13.9394, -13.1597) (-13.9494, -13.1489) (-13.9594, -13.1382) (-13.9696, -13.1275) (-13.9798, -13.1168) (-13.99, -13.1061) (-14.0004, -13.0955) (-14.0108, -13.0849) (-14.0213, -13.0744) (-14.0318, -13.0639) (-14.0425, -13.0535) (-14.0532, -13.043) (-14.064, -13.0326) (-14.0748, -13.0223) (-14.0857, -13.012) (-14.0967, -13.0017) (-14.1077, -12.9915) (-14.1189, -12.9813) (-14.13, -12.9711) (-14.1413, -12.961) (-14.1526, -12.9509) (-14.164, -12.9408) (-14.1754, -12.9308) (-14.1869, -12.9208) (-14.1985, -12.9109) (-14.2101, -12.9009) (-14.2218, -12.8911) (-14.2336, -12.8812) (-14.2454, -12.8714) (-14.2573, -12.8617) (-14.2668, -12.8539) (-14.274, -12.8481) (-14.2789, -12.8442) (-14.2813, -12.8423) knots 0 0 0 0 0 0 0.01428571 0.02857143 0.04285714 0.05714286 0.07142857 0.08571429 0.1 0.11428571 0.12857143 0.14285714 0.15714286 0.17142857 0.18571429 0.2 0.21428571 0.22857143 0.24285714 0.25714286 0.27142857 0.28571429 0.3 0.31428571 0.32857143 0.34285714 0.35714286 0.37142857 0.38571429 0.4 0.41428571 0.42857143 0.44285714 0.45714286 0.47142857 0.48571429 0.5 0.51428571 0.52857143 0.54285714 0.55714286 0.57142857 0.58571429 0.6 0.61428571 0.62857143 0.64285714 0.65714286 0.67142857 0.68571429 0.7 0.71428571 0.72857143 0.74285714 0.75714286 0.77142857 0.78571429 0.8 0.81428571 0.82857143 0.84285714 0.85714286 0.87142857 0.88571429 0.9 0.91428571 0.92857143 0.94285714 0.95714286 0.97142857 0.98571429 1 1 1 1 1 1
  arc A26 (-14.2813, -12.8423) -> (-14.6436, -12.9958) centre (-11.6741, -19.5) ccw